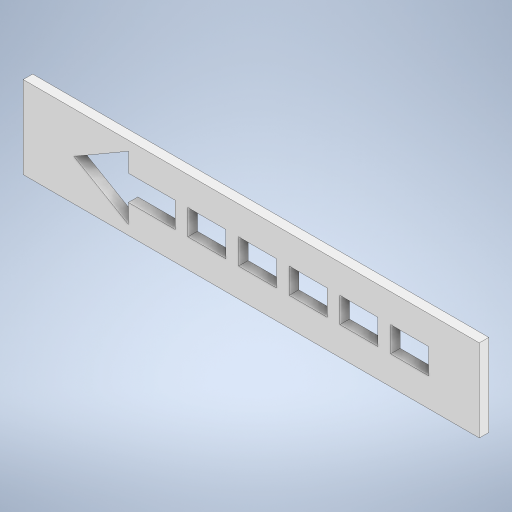
# Autodesk Inventor part: MS_R_Front_Green_v3
Saved by Autodesk Inventor 2024 (Build 280153000, 153)
## iProperties
Created: 2024-02-15
Part Number: MS_R_Front_Green_v3
Material: Generic
Document SubType Name: Modeling
Designer: LKLM
Density: 1 g/cm^3
Appearance: White
Author: LKLM
Autodesk Inventor part; units mm, degrees
ref_plane "YZ Plane" through (0, 0, 0) normal (1, 0, 0) x (0, 1, 0)
ref_plane "XZ Plane" through (0, 0, 0) normal (0, 1, 0) x (-1, 0, 0)
ref_plane "XY Plane" through (0, 0, 0) normal (0, 0, 1) x (1, 0, 0)
sketch "Sketch1" plane through (0, 0, 0) normal (0, 0, 1) x (1, 0, 0)
  line L0 (-64, 0) -> (-72, 0)
  line L1 (0, 37) -> (0, 24)
  line L2 (-72, 24) -> (-72, 37)
  line L3 (0, 0) -> (0, 24) construction
  line L4 (-72, 24) -> (0, 24)
  line L5 (-24, 22.0212) -> (-24, 32.5) construction
  line L6 (-24, 32.5) -> (-30, 32.5)
  line L7 (-30, 32.5) -> (-30, 28.5)
  line L8 (-30, 28.5) -> (-24, 28.5)
  line L9 (-24, 28.5) -> (-24, 32.5)
  line L10 (-30, 32.5) -> (-35, 32.5) construction
  line L11 (-22, 32.5) -> (-16, 32.5)
  line L12 (-16, 32.5) -> (-16, 28.5)
  line L13 (-16, 28.5) -> (-22, 28.5)
  line L14 (-22, 28.5) -> (-22, 32.5)
  line L15 (-14, 32.5) -> (-8, 32.5)
  line L16 (-8, 32.5) -> (-8, 28.5)
  line L17 (-8, 28.5) -> (-14, 28.5)
  line L18 (-14, 28.5) -> (-14, 32.5)
  line L19 (0, 24) -> (0, 37) construction
  line L20 (0, 37) -> (-91.064, 37) construction
  line L21 (0, 37) -> (-72, 37)
  line L22 (-72, 24) -> (-72, 37)
  line L23 (0, 24) -> (0, 37)
  line L24 (-72, 24) -> (-72, 30.5) construction
  line L25 (-72, 30.5) -> (-41.865, 30.5) construction
  line L26 (-64, 30.5) -> (-55.4, 30.5) construction
  line L27 (-55.4, 30.5) -> (-55.4, 35.5) construction
  line L28 (-55.4, 35.5) -> (-64, 30.5)
  line L29 (-55.4, 30.5) -> (-55.4, 25.5) construction
  line L30 (-64, 30.5) -> (-55.4, 25.5)
  line L31 (-32, 28.5) -> (-38, 28.5)
  line L32 (-38, 28.5) -> (-38, 32.5) construction
  line L33 (-38, 32.5) -> (-32, 32.5)
  line L34 (-32, 32.5) -> (-32, 28.5) construction
  line L35 (-38, 32.5) -> (-38, 28.5)
  line L36 (-32, 32.5) -> (-32, 28.5)
  line L37 (-40, 28.5) -> (-46, 28.5)
  line L38 (-46, 28.5) -> (-46, 32.5)
  line L39 (-46, 32.5) -> (-40, 32.5)
  line L40 (-40, 32.5) -> (-40, 28.5)
  line L41 (-55.4, 35.5) -> (-55.4, 32.5)
  line L42 (-55.4, 32.5) -> (-48, 32.5)
  line L43 (-48, 32.5) -> (-48, 28.5)
  line L44 (-48, 28.5) -> (-55.4, 28.5)
  line L45 (-55.4, 28.5) -> (-55.4, 25.5)
  point P0 (0, 0)
  point P1 (-137.4598, 47.0487)
  point P2 (-11, 28.5)
  point P3 (-11, 32.5)
  point P4 (-30, 30.5)
  point P5 (-32, 30.5)
  point P6 (-38, 30.5)
  point P7 (-40, 30.5)
  point P8 (-46, 30.5)
  point P9 (-48, 30.5)
  dimension "d3" = 0
  dimension "d4" = 0
  dimension "d8" = 24
  dimension "d14" = 6
  dimension "d19" = 6
  dimension "d20" = 4
  dimension "d21" = 6
  dimension "d22" = 2
  dimension "d23" = 2
  dimension "d33" = 8
  dimension "d36" = 28.5
  dimension "d37" = 13
  dimension "d38" = 4
  dimension "d39" = 8.6
  dimension "d40" = 5
  dimension "d41" = 5
  dimension "d42" = 6
  dimension "d43" = 4
  dimension "d44" = 2
  dimension "d45" = 6
  dimension "d46" = 2
  dimension "d47" = 3
  dimension "d48" = 7.4
  constraints: 92 end point, 12 parallel, 9 midpoint, 9 perpendicular, 8 horizontal, 6 collinear, 6 point on line, 2 vertical
  measures "d3" distance from line of L0 point (0, 0)
  measures "d4" distance from line of L1 point (0, 0)
  measures "d8" distance of L1.end L3.start
  measures "d14" distance of L8.end L7.end
  measures "d19" distance of L13.start L14.start
  measures "d20" distance of L11.end L13.start
  measures "d21" distance of L16.end L18.start
  measures "d22" distance between parallel lines of L9 L14
  measures "d23" distance between parallel lines of L12 L18
  measures "d33" distance from line of L16 point (0, 0)
  measures "d36" distance from line of L0 point (-11, 28.5)
  measures "d37" distance of L1.end L1.start
  measures "d38" distance from line of point (-11, 32.5) L17
  measures "d39" distance of L26.start L26.end
  measures "d40" distance of L26.end L27.end
  measures "d41" distance of L26.end L29.end
  measures "d42" distance of L32.end L33.end
  measures "d43" distance of L31.end L32.end
  measures "d44" distance of point (-30, 30.5) point (-32, 30.5)
  measures "d45" distance of L38.end L39.end
  measures "d46" distance of point (-38, 30.5) point (-40, 30.5)
  measures "d47" distance of L27.end L41.end
  measures "d48" distance of L41.end L42.end
extrude "Extrusion2" add sketch "Sketch1" along normal blind 1.5
body "Solid2"
